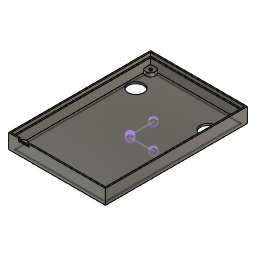
Case bottom (Autodesk Fusion 360 design; units mm, degrees)
Autodesk Fusion 360 part; units mm, degrees
sketch "PCB size" plane through (0, 0, 0) normal (0, 0, 1) x (1, 0, 0)
  line L0 (-40, 60) -> (40, 60)
  line L1 (40, 60) -> (40, -60)
  line L2 (40, -60) -> (-40, -60)
  line L3 (-40, -60) -> (-40, 60)
  line L4 (0, 1.75) -> (0, 22.5)
  line L5 (1.75, 0) -> (22.5, 0)
  dimension "d1" = 80
  dimension "d2" = 120
  constraint horizontal L0
  constraint vertical L1
  constraint horizontal L2
  constraint vertical L3
  constraint symmetric L0.start L0.end L4
  constraint symmetric L0.start L2.end L5
  measures "d1" distance of L0.start L0.end
  measures "d2" distance of L0.end L1.end
sketch "Space between PCB and wall" plane through (0, 0, 0) normal (0, 0, 1) x (1, 0, 0)
  line L0 (-40.5, 60.5) -> (40.5, 60.5)
  line L1 (40.5, 60.5) -> (40.5, -60.5)
  line L2 (40.5, -60.5) -> (-40.5, -60.5)
  line L3 (-40.5, -60.5) -> (-40.5, 60.5)
  point P0 (-40, 60)
  point P1 (40, 60)
  point P2 (40, -60)
  dimension "d3" = 0.5
  dimension "d4" = 0.5
  dimension "d5" = 0.5
  dimension "d6" = 0.5
  constraint horizontal L0
  constraint vertical L1
  constraint horizontal L2
  constraint vertical L3
  measures "d3" horizontal distance of L0.start P0
  measures "d4" horizontal distance of L0.end P1
  measures "d5" vertical distance of L0.end P1
  measures "d6" vertical distance of L1.end P2
extrude "Extrude1" add sketch "Space between PCB and wall" along normal blind 1.5
sketch "Wall" plane through (0, 0, 0) normal (0, 0, 1) x (1, 0, 0)
  line L0 (-42.9, -62.9) -> (42.9, -62.9)
  line L1 (42.9, -62.9) -> (42.9, 62.9)
  line L2 (42.9, 62.9) -> (-42.9, 62.9)
  line L3 (-42.9, 62.9) -> (-42.9, -62.9)
  line L4 (-40.5, 60.5) -> (40.5, 60.5)
  line L5 (40.5, 60.5) -> (40.5, -60.5)
  line L6 (40.5, -60.5) -> (-40.5, -60.5)
  line L7 (-40.5, -60.5) -> (-40.5, 60.5)
  point P0 (40.5, 60.5)
  point P1 (-40.5, 60.5)
  point P2 (-40.5, -60.5)
  dimension "d9" = 2.4
  dimension "d10" = 2.4
  dimension "d11" = 2.4
  dimension "d12" = 2.4
  constraint horizontal L0
  constraint vertical L1
  constraint horizontal L2
  constraint vertical L3
  constraint horizontal L4
  constraint vertical L5
  constraint horizontal L6
  constraint vertical L7
  constraint coincident P1 L4.start
  measures "d9" horizontal distance of L1.end P0
  measures "d10" horizontal distance of L2.end P1
  measures "d11" vertical distance of L0.start P2
  measures "d12" vertical distance of L2.end P1
extrude "Extrude2" add 1 faces at (-13.5, 20.1667, 1.5) along direction (0, 0, 1) blind 0.1
extrude "Extrude3" add sketch "Wall" along normal blind 13
sketch "Wall pad" plane through (0, 0, 13) normal (0, 0, 1) x (-1, 0, 0)
  line L0 (-40.5, 60.5) -> (40.5, 60.5)
  line L1 (40.5, 60.5) -> (40.5, -60.5)
  line L2 (40.5, -60.5) -> (-40.5, -60.5)
  line L3 (-40.5, -60.5) -> (-40.5, 60.5)
  line L4 (42.9, -62.9) -> (42.9, 62.9)
  line L5 (42.9, 62.9) -> (-42.9, 62.9)
  line L6 (-42.9, 62.9) -> (-42.9, -62.9)
  line L7 (-42.9, -62.9) -> (42.9, -62.9)
  line L8 (40.5, -60.5) -> (-40.5, -60.5)
  line L9 (-40.5, -60.5) -> (-40.5, 60.5)
  line L10 (-40.5, 60.5) -> (40.5, 60.5)
  line L11 (40.5, 60.5) -> (40.5, -60.5)
  line L12 (-41.7, 61.7) -> (41.7, 61.7)
  line L13 (41.7, 61.7) -> (41.7, -61.7)
  line L14 (41.7, -61.7) -> (-41.7, -61.7)
  line L15 (-41.7, -61.7) -> (-41.7, 61.7)
  dimension "d17" = 1.2
  dimension "d18" = 1.2
  dimension "d19" = 1.2
  dimension "d20" = 1.2
  constraint horizontal L8
  constraint vertical L9
  constraint horizontal L10
  constraint vertical L11
  constraint coincident L0.start L3.end
  constraint coincident L1.end L2.start
  constraint horizontal L12
  constraint vertical L13
  constraint horizontal L14
  constraint vertical L15
  measures "d17" horizontal distance of L1.end L13.end
  measures "d18" vertical distance of L1.end L13.end
  measures "d19" horizontal distance of L2.end L14.end
  measures "d20" vertical distance of L0.start L12.start
extrude "Extrude4" cut sketch "Wall pad" against normal blind 3 contours L12 L13 L14 L15
sketch "Screw holes" plane through (0, 0, 1.6) normal (0, 0, 1) x (-1, 0, 0)
  line L0 (40.5, 60.5) -> (-40.5, 60.5)
  line L1 (-40.5, 60.5) -> (-40.5, -60.5)
  line L2 (-40.5, -60.5) -> (40.5, -60.5)
  line L3 (40.5, -60.5) -> (40.5, 60.5)
  circle A0 centre (37, -57) radius 4.3
  circle A1 centre (-37, -57) radius 4.3
  circle A2 centre (-37, 57) radius 4.3
  circle A3 centre (37, 57) radius 4.3
  circle A4 centre (-37, -57) radius 1.1
  circle A5 centre (37, -57) radius 1.1
  circle A6 centre (37, 57) radius 1.1
  circle A7 centre (-37, 57) radius 1.1
  point P0 (40, -60)
  point P1 (37.0004, -61.3)
  point P2 (-40, -60)
  point P3 (-40, 60)
  point P4 (40, 60)
  dimension "d23" = 3
  dimension "d24" = 3
  dimension "d25" = 4.3
  dimension "d26" = 8.6
  dimension "d27" = 3
  dimension "d28" = 3
  dimension "d29" = 8.6
  dimension "d30" = 3
  dimension "d31" = 3
  dimension "d32" = 8.6
  dimension "d33" = 3
  dimension "d34" = 3
  dimension "d35" = 2.2
  dimension "d36" = 2.2
  dimension "d37" = 2.2
  dimension "d38" = 2.2
  constraint coincident A0 P1
  constraint concentric A1 A4
  constraint concentric A0 A5
  constraint concentric A3 A6
  constraint concentric A2 A7
  measures "d23" vertical distance of A0.centre P0
  measures "d24" horizontal distance of A0.centre P0
  measures "d25" vertical distance of A0.centre P1
  measures "d26" diameter of A1
  measures "d27" horizontal distance of A1.centre P2
  measures "d28" vertical distance of A1.centre P2
  measures "d29" diameter of A2
  measures "d30" horizontal distance of A2.centre P3
  measures "d31" vertical distance of A2.centre P3
  measures "d32" diameter of A3
  measures "d33" horizontal distance of A3.centre P4
  measures "d34" vertical distance of A3.centre P4
  measures "d35" diameter of A4
  measures "d36" diameter of A5
  measures "d37" diameter of A6
  measures "d38" diameter of A7
extrude "Extrude5" add sketch "Screw holes" along normal blind 3.2 contours L0 L3 A3 | L0 L1 A2 | L2 L3 A0 | L1 L2 A1 picked at (36.9726, 59.699) picked at (-36.9726, 59.699) picked at (36.9726, -59.699) picked at (-36.9726, -59.699)
thread "Thread1" "ISO Metric profile 2.5 M2.5x0.45 6H" major diameter 2.58 minor diameter 2.0755 pitch 0.45 angle 60 modelled right hand crest width 0.1211 on face at (35.9014, -56.9452, 3.7333) crest through (35.9622, -57, 1.7125) on face at (-38.0986, 57.0548, 3.7333) crest through (-38.0378, 57, 1.7125) on face at (35.9014, 57.0548, 3.7333) crest through (35.9622, 57, 1.7125) on face at (-38.0986, -56.9452, 3.7333) crest through (-38.0378, -57, 1.7125)
sketch "Leg holes" plane through (0, 0, 1.6) normal (0, 0, 1) x (-1, 0, 0)
  arc A0 (-34.502, -60.5) -> (-40.5, -54.502) centre (-37, -57) ccw
  line L0 (-34.502, -60.5) -> (34.502, -60.5)
  arc A1 (40.5, -54.502) -> (34.502, -60.5) centre (37, -57) ccw
  line L1 (40.5, -54.502) -> (40.5, 54.502)
  arc A2 (34.502, 60.5) -> (40.5, 54.502) centre (37, 57) ccw
  line L2 (34.502, 60.5) -> (-34.502, 60.5)
  arc A3 (-40.5, 54.502) -> (-34.502, 60.5) centre (-37, 57) ccw
  line L3 (-40.5, 54.502) -> (-40.5, -54.502)
  circle A4 centre (32, -39) radius 7
  circle A5 centre (-32, -39) radius 7
  point P0 (40, -60)
  point P1 (-40, -60)
  dimension "d41" = 14
  dimension "d42" = 21
  dimension "d43" = 8
  dimension "d44" = 14
  dimension "d45" = 8
  dimension "d46" = 21
  measures "d41" diameter of A4
  measures "d42" vertical distance of A4.centre P0
  measures "d43" horizontal distance of A4.centre P0
  measures "d44" diameter of A5
  measures "d45" horizontal distance of A5.centre P1
  measures "d46" vertical distance of A5.centre P1
extrude "Extrude6" cut sketch "Leg holes" against normal blind 1.6 contours A4 | A5
sketch "USB hole" plane through (0, -62.9, 0) normal (0, -1, 0) x (1, 0, 0)
  line L0 (-42.9, 0) -> (42.9, 0)
  line L1 (42.9, 0) -> (42.9, 13)
  line L2 (42.9, 13) -> (-42.9, 13)
  line L3 (-42.9, 13) -> (-42.9, 0)
  line L4 (-34, 13) -> (-24.9, 13)
  line L5 (-24.9, 13) -> (-24.9, 10.7)
  line L6 (-24.9, 10.7) -> (-34, 10.7)
  line L7 (-34, 10.7) -> (-34, 13)
  dimension "d49" = 8.9
  dimension "d50" = 2.3
  dimension "d51" = 9.1
  constraint horizontal L4
  constraint vertical L5
  constraint horizontal L6
  constraint vertical L7
  constraint coincident L2 L4.start
  measures "d49" distance of L2.end L4.start
  measures "d50" distance of L4.end L5.end
  measures "d51" distance of L4.start L4.end
extrude "Extrude7" cut sketch "USB hole" against normal blind 2.4 contours L2 L4 L5 L6 L7
equation "d26 = 4.3 * 2 mm"
named bodies: "Main"
